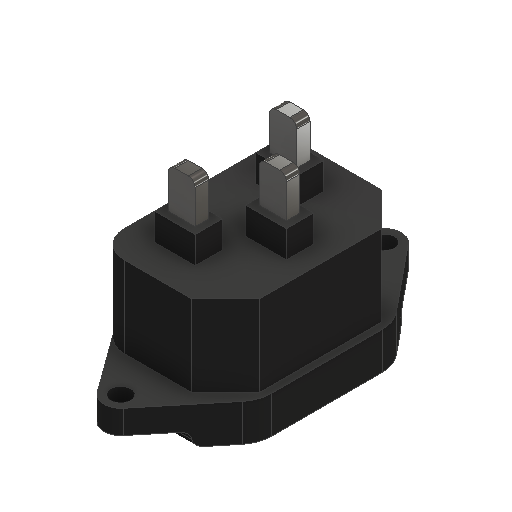
# Autodesk Inventor part: COTS_GENERIC_AC_Power_Socket_C14
Saved by Autodesk Inventor 2026.1 (Build 301233000, 233)
## iProperties
Created: 2016-06-24
Part Number: COTS_GENERIC_AC_Power_Socket_C14
Material: Ogólny
Document SubType Name: Modeling
Designer: Andrzej
Density: 1 g/cm^3
Appearance: Kauczuk - czarny
Mass: 4.71498 g
Surface Area: 51.3389 cm^2
Volume: 4.71498 cm^3
Author: Andrzej
Autodesk Inventor part; units mm, degrees
ref_plane "YZ Plane" through (0, 0, 0) normal (1, 0, 0) x (0, 1, 0)
ref_plane "XZ Plane" through (0, 0, 0) normal (0, 1, 0) x (-1, 0, 0)
ref_plane "XY Plane" through (0, 0, 0) normal (0, 0, 1) x (1, 0, 0)
sketch "Szkic1" plane through (0, 0, 0) normal (0, 0, 1) x (1, 0, 0)
  line L0 (-9.5177, 6.3249) -> (9.4823, 6.3249)
  line L1 (9.4823, 6.3249) -> (9.4823, -21.6751)
  line L2 (9.4823, -21.6751) -> (-9.5177, -21.6751)
  line L3 (-9.5177, -21.6751) -> (-9.5177, 6.3249)
  point P0 (0, 0)
  dimension "d0" = 19
  dimension "d1" = 28
  constraints: 8 end point, 2 parallel, 1 horizontal, 1 perpendicular
  measures "d0" distance of L1.end L2.end
  measures "d1" distance of L0.end L1.end
extrude "Wyciągnięcie proste1" add sketch "Szkic1" along normal blind 12
chamfer "Faza1" distance 5 angle 45 2 edges at (9.4823, 6.3249, 6) (9.4823, -21.6751, 6)
fillet "Zaokrąglenie1" radius 4 2 edges at (-9.5177, 6.3249, 6) (-9.5177, -21.6751, 6)
sketch "Szkic2" plane through (0, 0, 0) normal (0, 0, -1) x (-1, 0, 0)
  line L0 (-4.4823, -21.6751) -> (5.5177, -21.6751) projected
  line L1 (5.5177, 6.3249) -> (-4.4823, 6.3249) projected
  arc A0 (5.5177, -21.6751) -> (9.5177, -17.6751) centre (5.5177, -17.6751) ccw projected
  line L2 (9.5177, -17.6751) -> (9.5177, 2.3249) projected
  arc A1 (9.5177, 2.3249) -> (5.5177, 6.3249) centre (5.5177, 2.3249) ccw projected
  line L3 (5.5177, 6.3249) -> (-4.4823, 6.3249) projected
  line L4 (-9.4823, 1.3249) -> (-4.4823, 6.3249) projected
  line L5 (-9.4823, 1.3249) -> (-9.4823, -16.6751) projected
  line L6 (-4.4823, -21.6751) -> (-9.4823, -16.6751) projected
  line L7 (-4.4823, -21.6751) -> (5.5177, -21.6751) projected
  line L8 (7.5177, 2.3249) -> (7.5177, -17.6751)
  arc A2 (5.5177, -19.6751) -> (7.5177, -17.6751) centre (5.5177, -17.6751) ccw
  line L9 (5.5177, -19.6751) -> (-3.6539, -19.6751)
  line L10 (-3.6539, -19.6751) -> (-7.4823, -15.8467)
  line L11 (-7.4823, -15.8467) -> (-7.4823, 0.4965)
  line L12 (-7.4823, 0.4965) -> (-3.6539, 4.3249)
  line L13 (-3.6539, 4.3249) -> (5.5177, 4.3249)
  arc A3 (7.5177, 2.3249) -> (5.5177, 4.3249) centre (5.5177, 2.3249) ccw
  line L14 (10.5177, 2.3249) -> (10.5177, -17.6751)
  line L15 (-10.4823, 2.3249) -> (-10.4823, -17.6751)
  circle A4 centre (0.5177, 11.8249) radius 2.5
  circle A5 centre (0.5177, -27.1751) radius 2.5
  line L16 (-10.4823, -17.6751) -> (-1.4174, -28.7579)
  line L17 (10.5177, 2.3249) -> (2.5396, 13.2953)
  line L18 (10.5177, -17.6751) -> (2.5396, -28.6455)
  line L19 (-10.4823, 2.3249) -> (-1.4174, 13.4077)
  point P0 (0, 0)
  dimension "d8" = 28
  dimension "d9" = 2
  dimension "d10" = 20
  dimension "d11" = 1
  dimension "d12" = 4
  dimension "d13" = 20
  dimension "d14" = 1
  dimension "d15" = 4
  dimension "d16" = 10
  dimension "d17" = 10
  dimension "d18" = 39
  dimension "d19" = 5.5
  dimension "d20" = 5
  dimension "d21" = 5
  constraints: 24 end point, 8 point on circle, 4 centre point, 4 tangent, 2 coincident, 2 vertical, 7 other
  measures "d8" distance between parallel lines of L0 L1
  measures "d9" distance between parallel lines of L2 L8
  measures "d10" distance of L14.start L14.end
  measures "d11" distance between parallel lines of L2 L14
  measures "d12" distance from line of L14.start L1
  measures "d13" distance of L15.start L15.end
  measures "d14" distance between parallel lines of L5 L15
  measures "d15" distance from line of L1 L15.start
  measures "d16" distance from line of L14 point (0.518, -27.175)
  measures "d17" distance from line of L14 point (0.518, 11.825)
  measures "d18" distance of point (0.518, -27.175) point (0.518, 11.825)
  measures "d19" distance from line of point (0.518, -27.175) L0
  measures "d20" diameter of A4
  measures "d21" diameter of A5
extrude "Wyciągnięcie proste2" add sketch "Szkic2" along normal blind 5.5 contours L6 L5 L4 L1 A1 L2 A0 L0 | L14 L18 A5 L16 L15 L19 A4 L17 | A4 | A5
extrude "Wyciągnięcie proste3" cut sketch "Szkic2" against normal blind 11 contours L8 A2 L9 L10 L11 L12 L13 A3
hole "Otwór1" at (-0.5177, 11.8249, 0) at (-0.5177, -27.1751, 0) direction (0, 0, -1) diameter 3 end through all
sketch "Szkic3" plane through (0, 0, -5.5) normal (0, 0, -1) x (-1, 0, 0)
  circle A0 centre (0.5177, 11.8249) radius 1.5 projected
  circle A1 centre (0.5177, -27.1751) radius 1.5 projected
  arc A2 (5.5177, -19.6751) -> (7.5177, -17.6751) centre (5.5177, -17.6751) ccw projected
  line L0 (5.5177, -19.6751) -> (-3.6539, -19.6751) projected
  line L1 (-3.6539, -19.6751) -> (-7.4823, -15.8467) projected
  line L2 (-7.4823, -15.8467) -> (-7.4823, 0.4965) projected
  line L3 (-7.4823, 0.4965) -> (-3.6539, 4.3249) projected
  line L4 (-3.6539, 4.3249) -> (5.5177, 4.3249) projected
  arc A3 (7.5177, 2.3249) -> (5.5177, 4.3249) centre (5.5177, 2.3249) ccw projected
  line L5 (7.5177, 2.3249) -> (7.5177, -17.6751) projected
  arc A4 (-1.4174, -28.7579) -> (2.5396, -28.6455) centre (0.5177, -27.1751) ccw projected
  line L6 (2.5396, -28.6455) -> (10.5177, -17.6751) projected
  line L7 (10.5177, -17.6751) -> (10.5177, 2.3249) projected
  line L8 (10.5177, 2.3249) -> (2.5396, 13.2953) projected
  arc A5 (2.5396, 13.2953) -> (-1.4174, 13.4077) centre (0.5177, 11.8249) ccw projected
  line L9 (-1.4174, 13.4077) -> (-10.4823, 2.3249) projected
  line L10 (-10.4823, 2.3249) -> (-10.4823, -17.6751) projected
  line L11 (-10.4823, -17.6751) -> (-1.4174, -28.7579) projected
  line L12 (6.5179, 7.8249) -> (-5.9837, 7.8249)
  line L13 (6.5179, -23.1751) -> (-5.9837, -23.1751)
  point P0 (0, 0)
  dimension "d33" = 31
  dimension "d34" = 39
  dimension "d35" = 4
  constraints: 4 end point, 4 point on line, 2 horizontal
  measures "d33" distance between parallel lines of L13 L12
  measures "d34" distance of A1.centre A5.centre
  measures "d35" distance from line of A0.centre L12
extrude "Wyciągnięcie proste4" cut sketch "Szkic3" against normal blind 2 contours L11 L13 L6 A4 | L9 A5 L8 L12
fillet "Zaokrąglenie2" radius 1 4 edges at (-0.2671, 7.8249, -5.5) (-0.2671, 7.8249, -3.5) (-0.2671, -23.1751, -3.5) (-0.2671, -23.1751, -5.5)
fillet "Zaokrąglenie3" radius 5 4 edges at (-10.5177, 2.3249, -2.75) (-10.5177, -17.6751, -2.75) (10.4823, 2.3249, -2.75) (10.4823, -17.6751, -2.75)
sketch "Szkic4" plane through (0, 0, 11) normal (0, 0, -1) x (-1, 0, 0)
  line L0 (7.5177, 2.3249) -> (7.5177, -17.6751) projected
  arc A0 (7.5177, 2.3249) -> (5.5177, 4.3249) centre (5.5177, 2.3249) ccw projected
  line L1 (-3.6539, 4.3249) -> (5.5177, 4.3249) projected
  line L2 (-7.4823, 0.4965) -> (-3.6539, 4.3249) projected
  line L3 (-7.4823, -15.8467) -> (-7.4823, 0.4965) projected
  line L4 (-3.6539, -19.6751) -> (-7.4823, -15.8467) projected
  line L5 (5.5177, -19.6751) -> (-3.6539, -19.6751) projected
  arc A1 (5.5177, -19.6751) -> (7.5177, -17.6751) centre (5.5177, -17.6751) ccw projected
  line L6 (4.5177, 0.8249) -> (0.5177, 0.8249)
  line L7 (0.5177, 0.8249) -> (0.5177, -1.1751)
  line L8 (0.5177, -1.1751) -> (4.5177, -1.1751)
  line L9 (4.5177, -1.1751) -> (4.5177, 0.8249)
  line L10 (4.5177, -14.1751) -> (0.5177, -14.1751)
  line L11 (0.5177, -14.1751) -> (0.5177, -16.1751)
  line L12 (0.5177, -16.1751) -> (4.5177, -16.1751)
  line L13 (4.5177, -16.1751) -> (4.5177, -14.1751)
  line L14 (-1.4823, -6.6751) -> (-5.4823, -6.6751)
  line L15 (-5.4823, -6.6751) -> (-5.4823, -8.6751)
  line L16 (-5.4823, -8.6751) -> (-1.4823, -8.6751)
  line L17 (-1.4823, -8.6751) -> (-1.4823, -6.6751)
  point P0 (0, 0)
  dimension "d40" = 4
  dimension "d41" = 2
  dimension "d42" = 4
  dimension "d43" = 2
  dimension "d44" = 4
  dimension "d45" = 2
  dimension "d46" = 13
  dimension "d47" = 24
  dimension "d48" = 3.5
  dimension "d49" = 5.5
  dimension "d50" = 2
  dimension "d51" = 3
  dimension "d52" = 3
  constraints: 24 end point, 6 parallel, 3 horizontal, 3 perpendicular, 1 point on line
  measures "d40" distance of L8.end L7.end
  measures "d41" distance of L7.end L6.end
  measures "d42" distance of L12.end L11.end
  measures "d43" distance of L11.end L10.end
  measures "d44" distance of L16.end L15.end
  measures "d45" distance of L15.end L14.end
  measures "d46" distance between parallel lines of L10 L8
  measures "d47" distance between parallel lines of L1 L5
  measures "d48" distance between parallel lines of L1 L6
  measures "d49" distance between parallel lines of L14 L8
  measures "d50" distance between parallel lines of L7 L17
  measures "d51" distance between parallel lines of L0 L9
  measures "d52" distance between parallel lines of L0 L13
extrude "Wyciągnięcie proste5" add sketch "Szkic4" along normal blind 15 contours L9 L8 L7 L6 | L13 L12 L11 L10 | L17 L16 L15 L14
fillet "Zaokrąglenie4" radius 2 6 edges at (1.4823, -7.6751, -4) (5.4823, -7.6751, -4) (-0.5177, -0.1751, -4) (-4.5177, -0.1751, -4) (-0.5177, -15.1751, -4) (-4.5177, -15.1751, -4)
sketch "Szkic5" plane through (0, 0, 12) normal (0, 0, 1) x (1, 0, 0)
  arc A0 (-9.5177, -17.6751) -> (-5.5177, -21.6751) centre (-5.5177, -17.6751) ccw projected
  line L0 (-5.5177, -21.6751) -> (4.4823, -21.6751) projected
  line L1 (9.4823, -16.6751) -> (4.4823, -21.6751) projected
  line L2 (9.4823, -16.6751) -> (9.4823, 1.3249) projected
  line L3 (4.4823, 6.3249) -> (9.4823, 1.3249) projected
  line L4 (4.4823, 6.3249) -> (-5.5177, 6.3249) projected
  arc A1 (-5.5177, 6.3249) -> (-9.5177, 2.3249) centre (-5.5177, 2.3249) ccw projected
  line L5 (-9.5177, 2.3249) -> (-9.5177, -17.6751) projected
  line L6 (-0.5177, -14.1751) -> (-4.5177, -14.1751) projected
  line L7 (-4.5177, -16.1751) -> (-0.5177, -16.1751) projected
  line L8 (-4.5177, -14.1751) -> (-4.5177, -16.1751) projected
  line L9 (-0.5177, -16.1751) -> (-0.5177, -14.1751) projected
  line L10 (-4.5177, -1.1751) -> (-0.5177, -1.1751) projected
  line L11 (-0.5177, 0.8249) -> (-4.5177, 0.8249) projected
  line L12 (-4.5177, 0.8249) -> (-4.5177, -1.1751) projected
  line L13 (-0.5177, -1.1751) -> (-0.5177, 0.8249) projected
  line L14 (1.4823, -8.6751) -> (5.4823, -8.6751) projected
  line L15 (5.4823, -6.6751) -> (1.4823, -6.6751) projected
  line L16 (5.4823, -8.6751) -> (5.4823, -6.6751) projected
  line L17 (1.4823, -6.6751) -> (1.4823, -8.6751) projected
  line L18 (-5.5177, -17.1751) -> (0.4823, -17.1751)
  line L19 (0.4823, -17.1751) -> (0.4823, -13.1751)
  line L20 (0.4823, -13.1751) -> (-5.5177, -13.1751)
  line L21 (-5.5177, -13.1751) -> (-5.5177, -17.1751)
  line L22 (0.4823, -9.6751) -> (6.4823, -9.6751)
  line L23 (6.4823, -9.6751) -> (6.4823, -5.6751)
  line L24 (6.4823, -5.6751) -> (0.4823, -5.6751)
  line L25 (0.4823, -5.6751) -> (0.4823, -9.6751)
  line L26 (0.4823, 1.8249) -> (-5.5177, 1.8249)
  line L27 (-5.5177, 1.8249) -> (-5.5177, -2.1751)
  line L28 (-5.5177, -2.1751) -> (0.4823, -2.1751)
  line L29 (0.4823, -2.1751) -> (0.4823, 1.8249)
  point P0 (0, 0)
  dimension "d56" = 1
  dimension "d57" = 1
  dimension "d58" = 1
  constraints: 24 end point, 9 other
  measures "d56" distance between parallel lines of L8 L21
  measures "d57" distance between parallel lines of L17 L25
  measures "d58" distance between parallel lines of L13 L29
extrude "Wyciągnięcie proste6" add sketch "Szkic5" along normal blind 10 contours L9 L7 L8 L6 | L12 L11 L13 L10 | L17 L15 L16 L14
extrude "Wyciągnięcie proste7" add sketch "Szkic5" along normal blind 4 contours L21 L20 L19 L18 | L25 L24 L23 L22 | L29 L28 L27 L26
fillet "Zaokrąglenie5" radius 1 6 edges at (-4.5177, -15.1751, 22) (-0.5177, -15.1751, 22) (-4.5177, -0.1751, 22) (-0.5177, -0.1751, 22) (1.4823, -7.6751, 22) (5.4823, -7.6751, 22)
equation "\"d12\" = -0.5 * d10 + 0.5 * d8"
equation "\"d14\" = d11"
equation "\"d15\" = d12"
equation "\"d19\" = -0.5 * d8 + 0.5 * d18"
equation "\"d35\" = -0.5 * d33 + 0.5 * d34"
